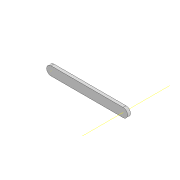
# Autodesk Inventor part: Recta_Theta1
Saved by Autodesk Inventor 2021 (Build 250183000, 183)
## iProperties
Created: 2021-07-18
Part Number: Recta_Theta1
Material: Generic
Document SubType Name: Modeling
Designer: Santiago
Density: 1 g/cm^3
Appearance: Default
Author: Santiago
Autodesk Inventor part; units mm, degrees
ref_plane "YZ Plane" through (0, 0, 0) normal (1, 0, 0) x (0, 1, 0)
ref_plane "XZ Plane" through (0, 0, 0) normal (0, 1, 0) x (-1, 0, 0)
ref_plane "XY Plane" through (0, 0, 0) normal (0, 0, 1) x (1, 0, 0)
sketch "Sketch1" plane through (0, 0, 0) normal (0, 0, 1) x (1, 0, 0)
  line L0 (0, 0) -> (245, 0)
  line L1 (0, 0) -> (245, 0) construction
  line L2 (0, -15) -> (245, -15)
  line L3 (245, 15) -> (0, 15)
  arc A0 (0, 15) -> (0, -15) centre (0, 0) ccw
  arc A1 (245, -15) -> (245, 15) centre (245, 0) ccw
  point P0 (122.5, 0)
  dimension "d1" = 245
  dimension "d2" = 30
  constraints: 10 end point, 4 point on circle, 4 tangent, 2 centre point, 2 equal length, 1 horizontal, 1 midpoint
  measures "d1" distance of L0.start L0.end
  measures "d2" diameter of A1
extrude "Extrusion1" add sketch "Sketch1" along normal blind 10
body "Solid1"
